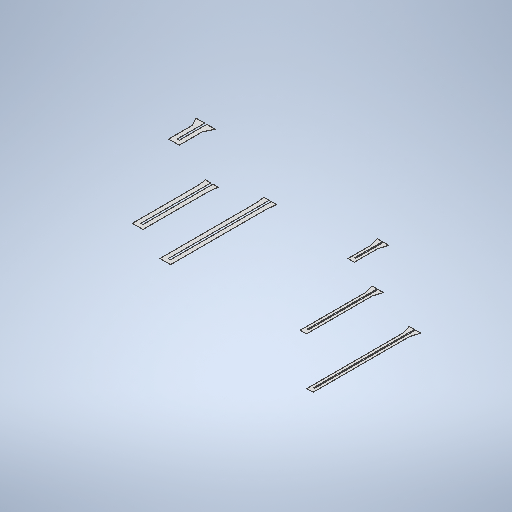
# Autodesk Inventor part: Design_Sensori
Saved by Autodesk Inventor 2025.4 (Build 294407000, 407)
## iProperties
Created: 2026-03-04
Part Number: Design_Sensori
Material: Generico
Document SubType Name: Modeling
Designer: Daniele
Density: 1 g/cm^3
Appearance: Default
Author: Daniele
Autodesk Inventor part; units mm, degrees
ref_plane "YZ Plane" through (0, 0, 0) normal (1, 0, 0) x (0, 1, 0)
ref_plane "XZ Plane" through (0, 0, 0) normal (0, 1, 0) x (-1, 0, 0)
ref_plane "XY Plane" through (0, 0, 0) normal (0, 0, 1) x (1, 0, 0)
sketch "Schizzo1" plane through (0, 0, 0) normal (0, 1, 0) x (-1, 0, 0)
  line L0 (-103.5, 44) -> (-103.5, -44)
  line L1 (-103.5, 44) -> (12.5, 44)
  line L2 (12.5, 44) -> (12.5, -44)
  line L3 (12.5, -44) -> (-103.5, -44)
  line L4 (-103.5, -44) -> (-103.5, 44)
  line L5 (96.5, 22) -> (12.5, 22)
  line L6 (-103.5, 44) -> (81.5, 44)
  line L7 (81.5, 44) -> (81.5, 22)
  line L8 (81.5, 0) -> (81.5, -22)
  line L9 (-103.5, -44) -> (60.5, -44)
  line L10 (60.5, -44) -> (60.5, -22)
  line L11 (96.5, 22) -> (96.5, 0)
  line L12 (81.5, -22) -> (60.5, -22)
  line L13 (12.5, -22) -> (60.5, -22)
  line L14 (96.5, 0) -> (12.5, 0)
  line L15 (-61.6109, -344.9655) -> (-55.6109, -344.9655)
  line L16 (-58.1109, -443.9655) -> (-58.1109, -348.9655)
  line L17 (-58.1109, -348.9655) -> (-59.1109, -348.9655)
  line L18 (-59.1109, -348.9655) -> (-59.1109, -443.9655)
  line L19 (-61.6109, -435.9655) -> (-64.1109, -443.9655)
  line L20 (-59.7734, -443.9655) -> (-64.1109, -443.9655)
  line L21 (-55.6109, -443.9655) -> (-53.1109, -443.9655)
  line L22 (-61.6109, -344.9655) -> (-61.6109, -435.9655)
  line L23 (-55.6109, -344.9655) -> (-55.6109, -435.9655)
  line L24 (-59.1109, -443.9655) -> (-59.7734, -443.9655)
  line L25 (-55.6109, -443.9655) -> (-58.1109, -443.9655)
  line L26 (-55.6109, -435.9655) -> (-53.1109, -443.9655)
  line L27 (109.9038, -381.9362) -> (119.9038, -381.9362)
  line L28 (115.9038, -480.9362) -> (115.9038, -385.9362)
  line L29 (115.9038, -385.9362) -> (113.9038, -385.9362)
  line L30 (113.9038, -385.9362) -> (113.9038, -480.9362)
  line L31 (109.9038, -472.9362) -> (108.9038, -480.9362)
  line L32 (113.2413, -480.9362) -> (108.9038, -480.9362)
  line L33 (118.4038, -480.9362) -> (120.9038, -480.9362)
  line L34 (109.9038, -381.9362) -> (109.9038, -472.9362)
  line L35 (119.9038, -381.9362) -> (119.9038, -472.9362)
  line L36 (113.9038, -480.9362) -> (113.2413, -480.9362)
  line L37 (118.4038, -480.9362) -> (115.9038, -480.9362)
  line L38 (119.9038, -472.9362) -> (120.9038, -480.9362)
  line L39 (-10.8405, -389.4949) -> (-4.8405, -389.4949)
  line L40 (-7.3405, -459.4949) -> (-7.3405, -393.4949)
  line L41 (-7.3405, -393.4949) -> (-8.3405, -393.4949)
  line L42 (-8.3405, -393.4949) -> (-8.3405, -459.4949)
  line L43 (-10.8405, -451.4949) -> (-13.3405, -459.4949)
  line L44 (-9.0029, -459.4949) -> (-13.3405, -459.4949)
  line L45 (-4.8405, -459.4949) -> (-2.3405, -459.4949)
  line L46 (-10.8405, -389.4949) -> (-10.8405, -451.4949)
  line L47 (-4.8405, -389.4949) -> (-4.8405, -451.4949)
  line L48 (-8.3405, -459.4949) -> (-9.0029, -459.4949)
  line L49 (-4.8405, -459.4949) -> (-7.3405, -459.4949)
  line L50 (-4.8405, -451.4949) -> (-2.3405, -459.4949)
  line L51 (25.1974, -470.6087) -> (31.1974, -470.6087)
  line L52 (28.6974, -500.6087) -> (28.6974, -474.6087)
  line L53 (28.6974, -474.6087) -> (27.6974, -474.6087)
  line L54 (27.6974, -474.6087) -> (27.6974, -500.6087)
  line L55 (25.1974, -492.6087) -> (22.6974, -500.6087)
  line L56 (27.0349, -500.6087) -> (22.6974, -500.6087)
  line L57 (31.1974, -500.6087) -> (33.6974, -500.6087)
  line L58 (25.1974, -470.6087) -> (25.1974, -492.6087)
  line L59 (31.1974, -470.6087) -> (31.1974, -492.6087)
  line L60 (27.6974, -500.6087) -> (27.0349, -500.6087)
  line L61 (31.1974, -500.6087) -> (28.6974, -500.6087)
  line L62 (31.1974, -492.6087) -> (33.6974, -500.6087)
  line L63 (151.6525, -397.6585) -> (161.6525, -397.6585)
  line L64 (157.6525, -401.6585) -> (155.6525, -401.6585)
  line L65 (160.1525, -467.6585) -> (162.6525, -467.6585)
  line L66 (161.6525, -459.6585) -> (162.6525, -467.6585)
  line L67 (160.1525, -467.6585) -> (157.6525, -467.6585)
  line L68 (155.6525, -467.6585) -> (154.99, -467.6585)
  line L69 (157.6525, -467.6585) -> (157.6525, -401.6585)
  line L70 (155.6525, -401.6585) -> (155.6525, -467.6585)
  line L71 (161.6525, -397.6585) -> (161.6525, -459.6585)
  line L72 (151.6525, -397.6585) -> (151.6525, -459.6585)
  line L73 (151.6525, -459.6585) -> (150.6525, -467.6585)
  line L74 (154.99, -467.6585) -> (150.6525, -467.6585)
  line L75 (203.39, -483.6182) -> (213.39, -483.6182)
  line L76 (209.39, -487.6182) -> (207.39, -487.6182)
  line L77 (211.89, -513.6182) -> (217.39, -513.6182)
  line L78 (213.39, -505.6182) -> (217.39, -513.6182)
  line L79 (211.89, -513.6182) -> (209.39, -513.6182)
  line L80 (207.39, -513.6182) -> (206.7275, -513.6182)
  line L81 (209.39, -513.6182) -> (209.39, -487.6182)
  line L82 (207.39, -487.6182) -> (207.39, -513.6182)
  line L83 (213.39, -483.6182) -> (213.39, -505.6182)
  line L84 (203.39, -483.6182) -> (203.39, -505.6182)
  line L85 (203.39, -505.6182) -> (199.39, -513.6182)
  line L86 (206.7275, -513.6182) -> (199.39, -513.6182)
  point P0 (0, 0)
  point P1 (-7.8405, -389.4949)
  point P2 (-7.8405, -393.4949)
  point P3 (-6.0905, -459.4949)
  point P4 (28.1974, -470.6087)
  point P5 (28.1974, -474.6087)
  point P6 (29.9474, -500.6087)
  point P7 (156.6525, -397.6585)
  point P8 (156.6525, -401.6585)
  point P9 (161.4025, -467.6585)
  point P10 (208.39, -483.6182)
  point P11 (208.39, -487.6182)
  point P12 (214.64, -513.6182)
  dimension "d2" = 116
  dimension "d3" = 185
  dimension "d4" = 164
  dimension "d5" = 200
  dimension "d18" = 5
  dimension "d19" = 1
  dimension "d20" = 2.5
  dimension "d21" = 5
  dimension "d22" = 2.5
  dimension "d23" = 5
  dimension "d26" = 5
  dimension "d29" = 4
  dimension "d30" = 4
  dimension "d32" = 2
  dimension "d35" = 5
  dimension "d36" = 1
  dimension "d37" = 2.5
  dimension "d38" = 5
  dimension "d39" = 2.5
  dimension "d40" = 4
  dimension "d41" = 70
  dimension "d42" = 5
  dimension "d43" = 1
  dimension "d44" = 2.5
  dimension "d45" = 5
  dimension "d46" = 2.5
  dimension "d47" = 4
  dimension "d48" = 30
  dimension "d49" = 5
  dimension "d50" = 5
  dimension "d51" = 4
  dimension "d52" = 4
  dimension "d53" = 2
  dimension "d54" = 4
  dimension "d55" = 70
  dimension "d56" = 8
  dimension "d57" = 8
  dimension "d58" = 4
  dimension "d59" = 4
  dimension "d60" = 2
  dimension "d61" = 4
  dimension "d62" = 30
  dimension "d63" = 6
  constraints: 174 end point, 21 perpendicular, 14 horizontal, 13 collinear, 13 midpoint, 10 point on line, 8 parallel, 2 vertical
  measures "d2" distance of L2.end L3.end
  measures "d3" distance of L0.start L6.end
  measures "d4" distance of L3.end L9.end
  measures "d5" distance between parallel lines of L0 L11
  measures "d18" distance of L21.end L16.start
  measures "d19" distance of L18.end L16.start
  measures "d20" distance between parallel lines of L16 L23
  measures "d21" distance of L19.end L18.end
  measures "d22" distance between parallel lines of L22 L18
  measures "d23" distance of L33.end L37.end
  measures "d26" distance of L31.end L36.start
  measures "d29" distance between parallel lines of L28 L35
  measures "d30" distance between parallel lines of L34 L30
  measures "d32" distance between parallel lines of L30 L28
  measures "d35" distance of L45.end L49.end
  measures "d36" distance of L42.end L49.end
  measures "d37" distance between parallel lines of L40 L47
  measures "d38" distance of L43.end L42.end
  measures "d39" distance between parallel lines of L46 L42
  measures "d40" distance of point (-7.84, -389.495) point (-7.84, -393.495)
  measures "d41" distance from line of L39 point (-6.09, -459.495)
  measures "d42" distance of L57.end L61.end
  measures "d43" distance of L54.end L61.end
  measures "d44" distance between parallel lines of L52 L59
  measures "d45" distance of L55.end L54.end
  measures "d46" distance between parallel lines of L58 L54
  measures "d47" distance of point (28.197, -470.609) point (28.197, -474.609)
  measures "d48" vertical distance of point (28.197, -470.609) point (29.947, -500.609)
  measures "d49" distance of L65.end L67.end
  measures "d50" distance of L73.end L68.start
  measures "d51" distance between parallel lines of L69 L71
  measures "d52" distance between parallel lines of L72 L70
  measures "d53" distance between parallel lines of L70 L69
  measures "d54" distance of point (156.653, -397.658) point (156.653, -401.658)
  measures "d55" distance from line of L63 point (161.403, -467.658)
  measures "d56" distance of L77.end L79.end
  measures "d57" distance of L85.end L80.start
  measures "d58" distance between parallel lines of L81 L83
  measures "d59" distance between parallel lines of L84 L82
  measures "d60" distance between parallel lines of L82 L81
  measures "d61" distance of point (208.39, -483.618) point (208.39, -487.618)
  measures "d62" distance from line of point (214.64, -513.618) L75
  measures "d63" distance between parallel lines of L58 L59
extrude "Estrusione1" add sketch "Schizzo1" along normal blind 0.15 contours L15 L23 L26 L21 L25 L16 L17 L18 L24 L20 L19 L22 | L27 L35 L38 L33 L37 L28 L29 L30 L36 L32 L31 L34 | L39 L47 L50 L45 L49 L40 L41 L42 L48 L44 L43 L46 | L51 L59 L62 L57 L61 L52 L53 L54 L60 L56 L55 L58 | L63 L71 L66 L65 L67 L69 L64 L70 L68 L74 L73 L72 | L75 L83 L78 L77 L79 L81 L76 L82 L80 L86 L85 L84
